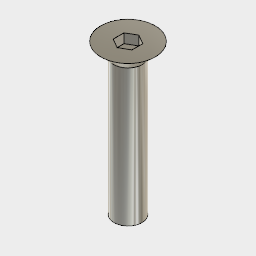
Bed_Surface_v3 (Autodesk Fusion 360 archive; units mm, degrees)
design "Bed Level Screw"
Autodesk Fusion 360 part; units mm, degrees
sketch "Body" plane through (0, 0, 0) normal (0, 1, 0) x (1, 0, 0) in component "Bed Level Screw"
  line L0 (-2.9, -16) -> (-0.8494, -16) construction
  line L1 (-2.9, -16) -> (-1.5, -14.6)
  line L2 (0, 0) -> (0, -16)
  line L3 (-1.5, -14.6) -> (-1.5, 0)
  line L4 (0, 0) -> (-1.5, 0)
  line L5 (0, -16) -> (-2.9, -16)
  dimension "d1" = 16
  dimension "d2" = 2.9
  dimension "d3" = 1.5
  dimension "d4" = 45
  measures "d1" distance of L2.start L2.end
  measures "d2" distance of L2.end L0.start
  measures "d3" distance of L3.end L2.start
  measures "d4" angle of L0 L1
revolve "Revolve1" add sketch "Body" angle 360 about axis through (0, 0, 0) along (0, 0, 1) in component "Bed Level Screw"
sketch "Sketch2" plane through (0, 0, 16) normal (0, 0, 1) x (-1, 0, 0) in component "Bed Level Screw"
  circle A0 centre (0, 0) radius 2.9
  line L0 (-1, -0.5774) -> (0, -1.1547)
  line L1 (0, -1.1547) -> (1, -0.5774)
  line L2 (1, -0.5774) -> (1, 0.5774)
  line L3 (1, 0.5774) -> (0, 1.1547)
  line L4 (0, 1.1547) -> (-1, 0.5774)
  line L5 (-1, 0.5774) -> (-1, -0.5774)
  dimension "d6" = 2
  measures "d6" distance of L0 L3
extrude "Extrude1" cut sketch "Sketch2" against normal blind 1 contours L0 L1 L2 L3 L4 L5 in component "Bed Level Screw"
component "Bed Level Screw" placed x (1, 0, 0) y (0, 1, 0) z (0, 0, 1) at (0, 0, 0)
equation "d2 = ( 5.8 / 2 ) * 1 mm"

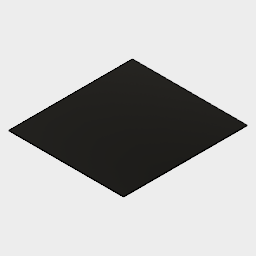
design "Print Surface"
Autodesk Fusion 360 part; units mm, degrees
sketch "Sketch1" plane through (0, 0, 0) normal (0, 0, 1) x (1, 0, 0) in component "Print Surface"
  line L0 (65, 70) -> (-65, 70)
  line L1 (-65, 70) -> (-65, -70)
  line L2 (-65, -70) -> (65, -70)
  line L3 (65, -70) -> (65, 70)
  line L4 (65, 70) -> (-65, -70) construction
  line L5 (-65, 70) -> (65, -70) construction
  dimension "d1" = 140
  dimension "d2" = 130
  measures "d1" distance of L0.end L1.end
  measures "d2" distance of L1.end L2.end
extrude "Extrude1" add sketch "Sketch1" along normal blind 0.5 in component "Print Surface"
component "Print Surface" placed x (1, 0, 0) y (0, 1, 0) z (0, 0, 1) at (0, 0, 0)

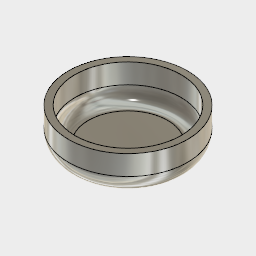
design "Bed Spring Cap"
Autodesk Fusion 360 part; units mm, degrees
sketch "Sketch1" plane through (0, 0, 0) normal (0, 1, 0) x (1, 0, 0) in component "Bed Spring Cap"
  arc A0 (4.5, -1.5) -> (3, 0) centre (3, -1.5) ccw
  arc A1 (-3, 0) -> (-4.5, -1.5) centre (-3, -1.5) ccw
  arc A2 (4, -1.5) -> (3, -0.5) centre (3, -1.5) ccw
  arc A3 (-3, -0.5) -> (-4, -1.5) centre (-3, -1.5) ccw
  line L0 (4.5, -1.5) -> (4.5, -3)
  line L1 (0, 0) -> (0, -0.5)
  line L2 (4, -3) -> (4.5, -3)
  line L3 (4, -1.5) -> (4, -3)
  line L4 (-3, -0.5) -> (3, -0.5)
  line L5 (-4, -3) -> (-4, -1.5)
  line L6 (-3, 0) -> (3, 0)
  line L7 (-4.5, -3) -> (-4, -3)
  line L8 (-4.5, -3) -> (-4.5, -1.5)
  dimension "d7" = 1.5
  dimension "d8" = 6
  dimension "d9" = 3
  dimension "d10" = 1
  dimension "d11" = 1.5
  measures "d7" radius of A0
  measures "d8" distance of A1.start A0.end
  measures "d9" distance of L7.start L6
  measures "d10" radius of A2
  measures "d11" distance of L7.start A1.end
revolve "Revolve1" add sketch "Sketch1" angle 360 about axis through (0, 0, 0) along (0, 0, 1) contours A1 A3 L1 L4 L5 L6 L7 L8 in component "Bed Spring Cap"
component "Bed Spring Cap" placed x (1, 0, 0) y (0, 1, 0) z (0, 0, 1) at (0, 0, 0)

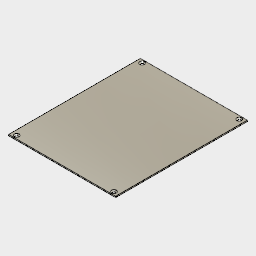
design "Heatbed"
Autodesk Fusion 360 part; units mm, degrees
sketch "Sketch1" plane through (0, 0, 0) normal (0, 0, 1) x (1, 0, 0) in component "Heatbed"
  line L0 (65, 80) -> (-65, 80)
  line L1 (-65, 80) -> (-65, -80)
  line L2 (-65, -80) -> (65, -80)
  line L3 (65, -80) -> (65, 80)
  line L4 (65, 0) -> (-89.1694, 0) construction
  line L5 (0, 80) -> (0, -80) construction
  circle A0 centre (-59, -76) radius 1.5
  circle A1 centre (59, -76) radius 1.5
  circle A2 centre (-59, 76) radius 1.5
  circle A3 centre (59, 76) radius 1.5
  dimension "d1" = 130
  dimension "d2" = 160
  dimension "d3" = 3
  dimension "d4" = 6
  dimension "d5" = 4
  measures "d1" distance of L1.end L2.end
  measures "d2" distance of L0.end L1.end
  measures "d3" diameter of A0
  measures "d4" distance of L1 A0.centre
  measures "d5" distance of L2 A0.centre
extrude "Extrude1" add sketch "Sketch1" along normal blind 1.5 in component "Heatbed"
chamfer "Chamfer1" distance 1.4 angle 45 4 edges at (-60.3985, 76.5424, 1.5) (57.6015, 76.5424, 1.5) (-60.3985, -75.4576, 1.5) (57.6015, -75.4576, 1.5) in component "Heatbed"
component "Heatbed" placed x (1, 0, 0) y (0, 1, 0) z (0, 0, 1) at (0, 0, 0)
